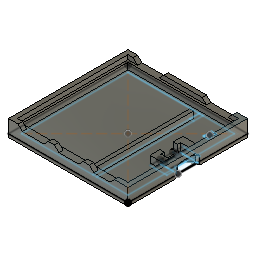
TesterHolder (Autodesk Fusion 360 design; units mm, degrees)
Autodesk Fusion 360 part; units mm, degrees
sketch "Sketch1" plane through (0, 0, 0) normal (0, 0, 1) x (1, 0, 0)
  line L0 (0, 0) -> (50, 0)
  line L1 (50, 0) -> (50, 50)
  line L2 (50, 50) -> (0, 50)
  line L3 (0, 50) -> (0, 0)
  dimension "d1" = 50
  dimension "d2" = 50
  constraint horizontal L0
  constraint vertical L1
  constraint horizontal L2
  constraint vertical L3
  constraint coincident L0.start L3.end
  measures "d1" distance of L0.start L0.end
  measures "d2" distance of L0.start L2.end
sketch "Sketch2" plane through (0, 0, 0) normal (0, 0, 1) x (1, 0, 0)
  line L0 (0, 50) -> (50, 0)
  line L1 (50.25, -0.25) -> (-0.25, -0.25)
  line L2 (-0.25, -0.25) -> (-0.25, 50.25)
  line L3 (-0.25, 50.25) -> (50.25, 50.25)
  line L4 (50.25, 50.25) -> (50.25, -0.25)
  line L5 (50.25, -0.25) -> (-0.25, 50.25) construction
  line L6 (-0.25, -0.25) -> (50.25, 50.25) construction
  line L7 (52.25, -2.25) -> (-2.25, -2.25)
  line L8 (-2.25, -2.25) -> (-2.25, 52.25)
  line L9 (-2.25, 52.25) -> (52.25, 52.25)
  line L10 (52.25, 52.25) -> (52.25, -2.25)
  line L11 (52.25, -2.25) -> (-2.25, 52.25) construction
  line L12 (-2.25, -2.25) -> (52.25, 52.25) construction
  line L13 (4.293, -0.25) -> (13.893, -0.25)
  line L14 (20.694, -0.25) -> (29.894, -0.25)
  line L15 (36.6037, -0.25) -> (44, -0.25)
  line L16 (4.2342, 50.25) -> (13.9, 50.25)
  line L17 (35.6828, 50.25) -> (45.5, 50.25)
  line L18 (18.0871, 50.25) -> (31.7, 50.25)
  point P0 (25, 25)
  point P1 (25, 25)
  dimension "d3" = 50.5
  dimension "d4" = 50.5
  dimension "d5" = 54.5
  dimension "d6" = 54.5
  dimension "d7" = 9.6
  dimension "d8" = 9.2
  constraint horizontal L1
  constraint perpendicular L1 L2
  constraint parallel L1 L3
  constraint parallel L2 L4
  constraint coincident L5 P1
  constraint coincident L6 P1
  constraint midpoint L0 P1
  constraint horizontal L7
  constraint perpendicular L7 L8
  constraint parallel L7 L9
  constraint parallel L8 L10
  constraint coincident L11 P1
  constraint coincident L12 P1
  constraint coincident P1 P0
  constraint coincident L1 L13.start
  constraint perpendicular L2 L13
  constraint coincident L1 L14.start
  constraint parallel L1 L14
  constraint coincident L1 L15.start
  constraint coincident L1 L15.end
  constraint coincident L3 L16.start
  constraint coincident L3 L16.end
  constraint coincident L3 L17.start
  constraint coincident L3 L17.end
  constraint coincident L3 L18.start
  constraint coincident L3 L18.end
  measures "d3" distance of L2.end L3.end
  measures "d4" distance of L1.end L2.end
  measures "d5" distance of L8.end L9.end
  measures "d6" distance of L7.end L8.end
  measures "d7" distance of L13.start L13.end
  measures "d8" distance of L14.start L14.end
extrude "Extrude1" add sketch "Sketch2" along normal blind 2
extrude "Extrude2" add 1 faces at (23.5647, -1.5833, 0) along direction (0, 0, -1) blind 4
sketch "Sketch3" plane through (0, 0, -4) normal (0, 0, -1) x (1, 0, 0)
  line L0 (-0.25, 0.25) -> (50.25, 0.25)
  line L1 (50.25, 0.25) -> (50.25, -50.25)
  line L2 (50.25, -50.25) -> (-0.25, -50.25)
  line L3 (-0.25, -50.25) -> (-0.25, 0.25)
  line L4 (-2.25, -52.25) -> (52.25, -52.25)
  line L5 (52.25, -52.25) -> (52.25, 2.25)
  line L6 (52.25, 2.25) -> (-2.25, 2.25)
  line L7 (-2.25, 2.25) -> (-2.25, -52.25)
  line L8 (52.25, 2.25) -> (-2.25, 2.25)
  line L9 (-2.25, 2.25) -> (-2.25, -52.25)
  line L10 (-2.25, -52.25) -> (52.25, -52.25)
  line L11 (52.25, -52.25) -> (52.25, 2.25)
  line L12 (52.25, -25) -> (52.25, -29.5)
  line L13 (52.25, -29.5) -> (52.25, -20.5)
  line L14 (52.25, -20.5) -> (44.55, -20.5)
  line L15 (44.55, -20.5) -> (44.55, -29.5)
  line L16 (44.55, -29.5) -> (52.25, -29.5)
  line L17 (52.25, -29.5) -> (52.25, -20.5)
  line L18 (44.55, -20.5) -> (48.55, -20.5)
  line L19 (48.55, -20.5) -> (48.55, -29.5)
  line L20 (48.55, -29.5) -> (44.55, -29.5)
  line L21 (44.55, -29.5) -> (44.55, -20.5)
  line L22 (48.55, -20.5) -> (48.55, -22.8)
  line L23 (48.55, -22.8) -> (52.25, -20.5)
  line L24 (48.55, -29.5) -> (48.55, -27.2)
  line L25 (48.55, -27.2) -> (52.25, -29.5)
  line L26 (44.55, -29.5) -> (50.25, -29.5)
  line L27 (50.25, -29.5) -> (50.25, -32.5)
  line L28 (50.25, -32.5) -> (44.55, -32.5)
  line L29 (44.55, -32.5) -> (44.55, -29.5)
  line L30 (44.55, -20.5) -> (50.25, -20.5)
  line L31 (50.25, -20.5) -> (50.25, -17.5)
  line L32 (50.25, -17.5) -> (44.55, -17.5)
  line L33 (44.55, -17.5) -> (44.55, -20.5)
  line L34 (44.55, -25) -> (44.55, -22)
  line L35 (44.55, -25) -> (44.55, -28)
  line L36 (44.55, -32.5) -> (42.55, -32.5)
  line L37 (42.55, -32.5) -> (42.55, -28)
  line L38 (42.55, -28) -> (44.55, -28)
  line L39 (44.55, -28) -> (44.55, -32.5)
  line L40 (44.55, -22) -> (42.55, -22)
  line L41 (42.55, -22) -> (42.55, -17.5)
  line L42 (42.55, -17.5) -> (44.55, -17.5)
  line L43 (44.55, -17.5) -> (44.55, -22)
  dimension "d13" = 4.5
  dimension "d14" = 7.7
  dimension "d15" = 4
  dimension "d16" = 2.3
  dimension "d17" = 2.3
  dimension "d22" = 3
  dimension "d23" = 3
  dimension "d24" = 3
  dimension "d25" = 3
  dimension "d26" = 2
  dimension "d27" = 2
  constraint horizontal L8
  constraint vertical L9
  constraint horizontal L10
  constraint vertical L11
  constraint coincident L4.start L7.end
  constraint coincident L5.end L6.start
  constraint midpoint L5 L12.start
  constraint parallel L5 L12
  constraint coincident L5 L13.end
  constraint parallel L5 L13
  constraint horizontal L14
  constraint vertical L15
  constraint horizontal L16
  constraint vertical L17
  constraint horizontal L18
  constraint vertical L19
  constraint horizontal L20
  constraint vertical L21
  constraint perpendicular L14 L22
  constraint perpendicular L20 L24
  constraint horizontal L26
  constraint vertical L27
  constraint horizontal L28
  constraint vertical L29
  constraint horizontal L30
  constraint vertical L31
  constraint horizontal L32
  constraint vertical L33
  constraint midpoint L15 L34.start
  constraint perpendicular L18 L34
  constraint parallel L15 L35
  constraint horizontal L36
  constraint vertical L37
  constraint horizontal L38
  constraint vertical L39
  constraint horizontal L40
  constraint vertical L41
  constraint horizontal L42
  constraint vertical L43
  measures "d13" distance of L12.start L12.end
  measures "d14" distance of L13.end L14.end
  measures "d15" distance of L14.end L18.end
  measures "d16" distance of L18.end L22.end
  measures "d17" distance of L19.end L24.end
  measures "d22" distance of L15.end L28.end
  measures "d23" distance of L14.end L32.end
  measures "d24" distance of L34.start L34.end
  measures "d25" distance of L34.start L35.end
  measures "d26" distance of L28.end L36.end
  measures "d27" distance of L34.end L40.end
extrude "Extrude3" cut sketch "Sketch3" against normal blind 4 contours L1 L5 L11 L12 L13 L17 L23 L25
extrude "Extrude4" add sketch "Sketch3" along normal blind 1.5 contours L0 L1 L2 L3 L4 L5 L6 L7 L8 L9 L10 L11 L14 L16 L27 L31 | L0 L1 L2 L3 L15 L21 L28 L32 L34 L35 L36 L37 L38 L40 L41 L42 | L1 L14 L18 L30 L31 L32 L33 L43 | L1 L14 L23 | L1 L14 L19 L22 L23 L30 | L15 L21 L33 L40 L41 L42 L43 | L1 L16 L20 L26 L27 L28 L29 L39 | L14 L15 L16 L18 L19 L20 L21 L22 L24 L26 L30 L34 L35 L39 L43 | L1 L16 L19 L24 L25 L26 | L1 L16 L25 | L15 L21 L29 L36 L37 L38 L39
extrude "Extrude5" add sketch "Sketch3" against normal blind 4 contours L1 L14 L18 L30 L31 L32 L33 L43 | L1 L14 L19 L22 L23 L30 | L15 L21 L33 L40 L41 L42 L43 | L1 L16 L20 L26 L27 L28 L29 L39 | L1 L16 L19 L24 L25 L26 | L15 L21 L29 L36 L37 L38 L39
sketch "Sketch4" plane through (0, 0, -4) normal (0, 0, 1) x (-1, 0, 0)
  line L0 (-50.25, -17.5) -> (-42.55, -17.5)
  line L1 (-42.55, -17.5) -> (-42.55, -22)
  line L2 (-42.55, -22) -> (-44.55, -22)
  line L3 (-44.55, -22) -> (-44.55, -20.5)
  line L4 (-44.55, -20.5) -> (-48.55, -20.5)
  line L5 (-48.55, -20.5) -> (-48.55, -22.8)
  line L6 (-48.55, -22.8) -> (-48.55, -27.2)
  line L7 (-48.55, -27.2) -> (-48.55, -29.5)
  line L8 (-48.55, -29.5) -> (-44.55, -29.5)
  line L9 (-44.55, -29.5) -> (-44.55, -28)
  line L10 (-44.55, -28) -> (-42.55, -28)
  line L11 (-42.55, -28) -> (-42.55, -32.5)
  line L12 (-42.55, -32.5) -> (-50.25, -32.5)
  line L13 (-50.25, -32.5) -> (-50.25, -50.25)
  line L14 (-50.25, -50.25) -> (0.25, -50.25)
  line L15 (0.25, -50.25) -> (0.25, 0.25)
  line L16 (0.25, 0.25) -> (-50.25, 0.25)
  line L17 (-50.25, 0.25) -> (-50.25, -17.5)
  line L18 (-49.25, -0.75) -> (-0.75, -0.75)
  line L19 (-0.75, -0.75) -> (-0.75, -49.25)
  line L20 (-0.75, -49.25) -> (-49.25, -49.25)
  line L21 (-49.25, -49.25) -> (-49.25, -0.75)
  line L22 (-49.25, -0.75) -> (-0.75, -49.25) construction
  line L23 (-0.75, -0.75) -> (-49.25, -49.25) construction
  line L24 (-0.75, -49.25) -> (-33.25, -49.25)
  line L25 (-33.25, -49.25) -> (-33.25, -0.75)
  line L26 (-33.25, -49.25) -> (-35, -49.25)
  line L27 (-35, -49.25) -> (-35, -0.75)
  line L28 (-33.25, -49.25) -> (-33.25, -45)
  line L29 (-33.25, -45) -> (-35, -45)
  line L30 (-42.55, -28) -> (-42.55, -22)
  line L31 (-44.55, -28) -> (-44.55, -22)
  point P0 (-25, -25)
  dimension "d30" = 48.5
  dimension "d31" = 48.5
  dimension "d34" = 32.5
  constraint horizontal L18
  constraint perpendicular L18 L19
  constraint parallel L18 L20
  constraint parallel L19 L21
  constraint coincident L22 P0
  constraint coincident L23 P0
  constraint perpendicular L19 L24
  constraint coincident L18 L25.end
  constraint perpendicular L18 L25
  constraint coincident L20 L26.end
  constraint coincident L18 L27.end
  constraint perpendicular L18 L27
  constraint coincident L25 L28.end
  constraint coincident L27 L29.end
  constraint perpendicular L27 L29
  constraint coincident L10.end L11.start
  constraint coincident L1.end L2.start
  constraint coincident L9.end L10.start
  constraint coincident L2.end L3.start
  measures "d30" distance of L19.end L20.end
  measures "d31" distance of L18.end L19.end
  measures "d34" distance of L19.end L24.end
extrude "Extrude6" add sketch "Sketch4" along normal blind 4 contours L0 L12 L13 L14 L15 L16 L17 L18 L19 L20 L21 L24 L26
extrude "Extrude7" add sketch "Sketch4" along normal blind 4 contours L18 L25 L27 L29
extrude "Extrude8" add sketch "Sketch4" along normal blind 1 contours L0 L1 L11 L12 L18 L20 L21 L27 L30 | L20 L25 L26 L27 L28 L29 | L18 L19 L20 L24 L25 L28
extrude "Extrude9" add sketch "Sketch4" along normal blind 1 contours L2 L10 L30 L31
fillet "Fillet1" radius 1.5 9 edges at (52.25, 20.5, -2.75) (48.55, 22.8, -4.75) (48.55, 27.2, -4.75) (52.25, 29.5, -2.75) (51.25, 28.8784, 0) (51.25, 21.1216, 0) (50.4, 21.65, -5.5) (48.55, 25, -5.5) (50.4, 28.35, -5.5)
sketch "Sketch5" plane through (0, 0, 2) normal (0, 0, 1) x (-1, 0, 0)
  line L0 (-50.25, 0.25) -> (0.25, 0.25)
  line L1 (0.25, 0.25) -> (0.25, -50.25)
  line L2 (0.25, -50.25) -> (-50.25, -50.25)
  line L3 (-50.25, -50.25) -> (-50.25, 0.25)
  line L4 (-52.25, -52.25) -> (2.25, -52.25)
  line L5 (2.25, -52.25) -> (2.25, 2.25)
  line L6 (2.25, 2.25) -> (-52.25, 2.25)
  line L7 (-52.25, 2.25) -> (-52.25, -52.25)
  line L8 (-4.0784, 0.25) -> (-13.8889, 0.25)
  line L9 (-13.8889, 0.25) -> (-13.8889, 2.25)
  line L10 (-13.8889, 2.25) -> (-4.0784, 2.25)
  line L11 (-4.0784, 2.25) -> (-4.0784, 0.25)
  line L12 (-20.6651, 0.25) -> (-29.7986, 0.25)
  line L13 (-29.7986, 0.25) -> (-29.7986, 2.25)
  line L14 (-29.7986, 2.25) -> (-20.6651, 2.25)
  line L15 (-20.6651, 2.25) -> (-20.6651, 0.25)
  line L16 (-36.6346, 0.25) -> (-43.9893, 0.25)
  line L17 (-43.9893, 0.25) -> (-43.9893, 2.25)
  line L18 (-43.9893, 2.25) -> (-36.6346, 2.25)
  line L19 (-36.6346, 2.25) -> (-36.6346, 0.25)
  line L20 (-4.0784, -50.25) -> (-14.0527, -50.25)
  line L21 (-14.0527, -50.25) -> (-14.0527, -52.25)
  line L22 (-14.0527, -52.25) -> (-4.0784, -52.25)
  line L23 (-4.0784, -52.25) -> (-4.0784, -50.25)
  line L24 (-18.1744, -50.25) -> (-31.738, -50.25)
  line L25 (-31.738, -50.25) -> (-31.738, -52.25)
  line L26 (-31.738, -52.25) -> (-18.1744, -52.25)
  line L27 (-18.1744, -52.25) -> (-18.1744, -50.25)
  line L28 (-35.5568, -50.25) -> (-45.3767, -50.25)
  line L29 (-45.3767, -50.25) -> (-45.3767, -52.25)
  line L30 (-45.3767, -52.25) -> (-35.5568, -52.25)
  line L31 (-35.5568, -52.25) -> (-35.5568, -50.25)
  constraint horizontal L8
  constraint vertical L9
  constraint horizontal L10
  constraint vertical L11
  constraint coincident L6 L9.end
  constraint coincident L0 L8.start
  constraint horizontal L12
  constraint vertical L13
  constraint horizontal L14
  constraint vertical L15
  constraint coincident L6 L13.end
  constraint coincident L0 L12.start
  constraint horizontal L16
  constraint vertical L17
  constraint horizontal L18
  constraint vertical L19
  constraint coincident L6 L17.end
  constraint coincident L0 L16.start
  constraint horizontal L20
  constraint vertical L21
  constraint horizontal L22
  constraint vertical L23
  constraint coincident L4 L21.end
  constraint coincident L2 L20.start
  constraint horizontal L24
  constraint vertical L25
  constraint horizontal L26
  constraint vertical L27
  constraint coincident L4 L25.end
  constraint coincident L2 L24.start
  constraint horizontal L28
  constraint vertical L29
  constraint horizontal L30
  constraint vertical L31
  constraint coincident L4 L29.end
  constraint coincident L2 L28.start
extrude "Extrude10" cut sketch "Sketch5" against normal blind 2 contours L0 L6 L16 L17 L18 L19 | L2 L4 L28 L29 L30 L31 | L0 L6 L12 L13 L14 L15 | L0 L6 L8 L9 L10 L11 | L2 L4 L20 L21 L22 L23
chamfer "Chamfer1" distance 2 angle 45 1 edges at (4.0784, -1.25, 2)
chamfer "Chamfer2" distance 2 angle 45 5 edges at (13.8889, -1.25, 2) (20.6651, -1.25, 2) (29.7986, -1.25, 2) (36.6346, -1.25, 2) (43.9893, -1.25, 2)
chamfer "Chamfer3" distance 2 angle 45 4 edges at (45.3767, 51.25, 2) (35.5568, 51.25, 2) (14.0527, 51.25, 2) (4.0784, 51.25, 2)
sketch "Sketch6" plane through (0, 0, 2) normal (0, 0, 1) x (-1, 0, 0)
  line L0 (-47.3767, -52.25) -> (-47.3767, -50.25)
  line L1 (-47.3767, -50.25) -> (-50.25, -50.25)
  line L2 (-50.25, -50.25) -> (-50.25, 0.25)
  line L3 (-50.25, 0.25) -> (-45.9893, 0.25)
  line L4 (-45.9893, 0.25) -> (-45.9893, 2.25)
  line L5 (-45.9893, 2.25) -> (-52.25, 2.25)
  line L6 (-52.25, 2.25) -> (-52.25, -52.25)
  line L7 (-52.25, -52.25) -> (-47.3767, -52.25)
  line L8 (-51.3046, -35.3037) -> (-49.1954, -35.3037)
  line L9 (-49.1954, -35.3037) -> (-49.1954, -38.8722)
  line L10 (-49.1954, -38.8722) -> (-51.3046, -38.8722)
  line L11 (-51.3046, -38.8722) -> (-51.3046, -35.3037)
  line L12 (-51.3046, -35.3037) -> (-49.1954, -38.8722) construction
  line L13 (-49.1954, -35.3037) -> (-51.3046, -38.8722) construction
  point P0 (-50.25, -37.088)
  constraint horizontal L8
  constraint perpendicular L8 L9
  constraint parallel L8 L10
  constraint parallel L9 L11
  constraint coincident L12 P0
  constraint coincident L13 P0
  constraint coincident L2 P0
extrude "Extrude11" cut sketch "Sketch6" against normal blind 4 contours L2 L8 L10 L11
extrude "Extrude12" cut sketch "Sketch6" against normal blind 4 contours L2 L8 L9 L10
chamfer "Chamfer4" distance 1 angle 45 3 edges at (49.25, 38.8722, -1) (49.25, 37.088, -2) (49.25, 35.3037, -1)
